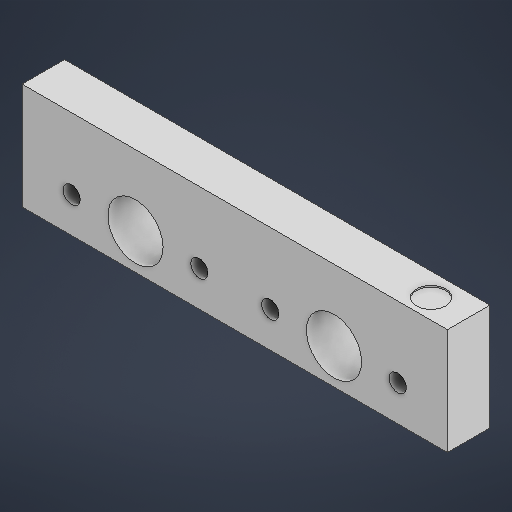
# Autodesk Inventor part: backmidmotorwall
Saved by Autodesk Inventor 2026.2 (Build 302298010, 298A)
## iProperties
Created: 2026-03-30
Part Number: backmidmotorwall
Material: Generic
Document SubType Name: Modeling
Designer: karol
Density: 1 g/cm^3
Appearance: Default
Author: karol
Autodesk Inventor part; units mm, degrees
ref_plane "YZ Plane" through (0, 0, 0) normal (1, 0, 0) x (0, 1, 0)
ref_plane "XZ Plane" through (0, 0, 0) normal (0, 1, 0) x (-1, 0, 0)
ref_plane "XY Plane" through (0, 0, 0) normal (0, 0, 1) x (1, 0, 0)
sketch "Sketch1" plane through (0, 0, 0) normal (0, 1, 0) x (-1, 0, 0)
  line L0 (0, 0) -> (30, 0)
  line L1 (30, 0) -> (30, -3)
  line L2 (30, -3) -> (0, -3)
  line L3 (0, -3) -> (0, 0)
  dimension "d0" = 30
  dimension "d1" = 3
  constraints: 8 end point, 2 parallel, 1 horizontal, 1 perpendicular
  measures "d0" distance of L1.end L2.end
  measures "d1" distance of L0.end L1.end
extrude "Extrusion1" add sketch "Sketch1" along normal blind 7.5
sketch "Sketch2" plane through (0, 7.5, 0) normal (0, 1, 0) x (1, 0, 0)
  circle A0 centre (-2.5481, 1.391) radius 1.0387
  point P0 (0, 0)
  constraints: 1 centre point
extrude "Extrusion2" cut sketch "Sketch2" against normal blind 0.1
sketch "Sketch3" plane through (-30, 0, 0) normal (0, 0, 1) x (1, 0, 0)
  circle A0 centre (26.5, 2.5) radius 0.6105
  line L0 (0, 0) -> (30, 0) projected
  line L1 (30, 0) -> (30, 7.5) projected
  circle A1 centre (22, 2.5) radius 1.95
  circle A2 centre (17.5, 2.5) radius 0.6105
  line L2 (30, 7.5) -> (0, 7.5) projected
  line L3 (0, 7.5) -> (30, 7.5)
  line L4 (30, 7.5) -> (15, 7.5)
  line L5 (15, 7.5) -> (15, 0)
  circle A3 centre (3.5, 2.5) radius 0.6105
  circle A4 centre (8, 2.5) radius 1.95
  circle A5 centre (12.5, 2.5) radius 0.6105
  dimension "d6" = 1.221
  dimension "d7" = 2.5
  dimension "d8" = 3.5
  dimension "d9" = 3.9
  dimension "d10" = 8
  dimension "d11" = 1.221
  dimension "d12" = 2.5
  dimension "d13" = 4.5
  constraints: 6 centre point, 6 end point, 3 symmetric about line, 2 midpoint, 1 collinear, 3 other
  measures "d6" diameter of A0
  measures "d7" distance from line of L0 A0.centre
  measures "d8" distance from line of L1 A0.centre
  measures "d9" diameter of A1
  measures "d10" distance from line of L1 A1.centre
  measures "d11" diameter of A2
  measures "d12" distance from line of L0 A2.centre
  measures "d13" distance of A1.centre A2.centre
extrude "Extrusion3" cut sketch "Sketch3" against normal blind 3 contours A0 | A1 | A2 | A3 | A4 | A5
body "Solid1"
